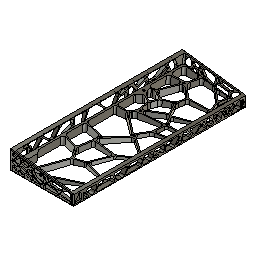
KEYBOARD CASE HOLY60 v20 - reduced size (Autodesk Fusion 360 design; units mm, degrees)
Autodesk Fusion 360 part; units mm, degrees
(part 1 of 5)
sketch "Sketch1" plane through (0, 0, 0) normal (0, 0, 1) x (1, 0, 0)
sketch "Bottom_Master" plane through (0, 0, 0) normal (0, 0, 1) x (1, 0, 0)
  line L0 (-6.9, 1.5441) -> (3.17, 1.5441)
  line L1 (3.17, 1.5441) -> (3.17, -2.18)
  line L2 (3.17, -2.18) -> (-6.9, -2.18)
  line L3 (-6.9, -2.18) -> (-6.9, 1.5441)
  line L4 (-6.7006, 1.3231) -> (2.9594, 1.3231)
  line L5 (3.0344, 1.2481) -> (3.0344, -1.9174)
  line L6 (2.9594, -1.9924) -> (-6.7006, -1.9924)
  line L7 (-6.7756, -1.9174) -> (-6.7756, 1.2481)
  line L8 (-6.6737, 0.97) -> (-6.6737, 0.6805)
  line L9 (-6.5896, 0.566) -> (-4.9141, 0.0417)
  line L10 (-4.8122, 0.054) -> (-4.3386, 0.3395)
  line L11 (-4.2652, 0.4409) -> (-4.1196, 1.0786)
  line L12 (-4.2463, 1.2375) -> (-5.5724, 1.2375)
  line L13 (-5.7409, 1.085) -> (-6.5587, 1.085)
  line L14 (-6.6737, 0.3825) -> (-6.6737, 0.3136)
  line L15 (-6.6459, 0.2188) -> (-5.3035, -1.8653)
  line L16 (-5.2194, -1.9111) -> (-4.9455, -1.9111)
  line L17 (-4.8222, -1.8065) -> (-4.628, -0.634)
  line L18 (-4.6398, -0.5466) -> (-4.8436, -0.1054)
  line L19 (-4.935, -0.0251) -> (-6.5439, 0.4779)
  line L20 (-6.5487, -1.9111) -> (-5.583, -1.9111)
  line L21 (-5.4781, -1.7181) -> (-6.4898, -0.1565)
  line L22 (-6.6737, -0.2109) -> (-6.6737, -1.7861)
  line L23 (-4.0329, 1.1248) -> (-4.1711, 0.5196)
  line L24 (-4.0646, 0.3677) -> (-3.11, 0.249)
  line L25 (-2.9431, 0.3758) -> (-2.8362, 1.0941)
  line L26 (-2.9598, 1.2375) -> (-3.8915, 1.2375)
  line L27 (-3.3566, 0.1098) -> (-3.372, -0.8279)
  line L28 (-3.5043, -0.9209) -> (-4.4494, -0.5985)
  line L29 (-4.5941, -0.4701) -> (-4.7474, -0.1509)
  line L30 (-4.6899, 0.0422) -> (-4.3293, 0.2609)
  line L31 (-4.1257, 0.3051) -> (-3.4581, 0.2259)
  line L32 (-4.7377, -1.7366) -> (-4.5829, -0.8022)
  line L33 (-4.386, -0.6849) -> (-3.406, -1.0231)
  line L34 (-3.3306, -1.0741) -> (-2.7509, -1.7458)
  line L35 (-2.8266, -1.9111) -> (-4.5897, -1.9111)
  line L36 (-3.2843, 0.055) -> (-3.3074, -0.9017)
  line L37 (-3.2468, -1.0711) -> (-2.7111, -1.6917)
  line L38 (-2.5519, -1.6814) -> (-1.9832, -0.8174)
  line L39 (-2.0116, -0.6495) -> (-3.0673, 0.159)
  line L40 (-2.4221, -1.9111) -> (-0.9115, -1.9111)
  line L41 (-0.8171, -1.7781) -> (-1.0763, -1.038)
  line L42 (-1.2125, -0.883) -> (-1.6826, -0.6472)
  line L43 (-1.8114, -0.6822) -> (-2.506, -1.7568)
  line L44 (-2.7588, 1.1526) -> (-2.8964, 0.2481)
  line L45 (-2.8298, 0.0829) -> (-2.0545, -0.5108)
  line L46 (-1.844, -0.4826) -> (-1.0421, 0.5699)
  line L47 (-1.0128, 0.6809) -> (-1.0765, 1.151)
  line L48 (-1.1756, 1.2375) -> (-2.6599, 1.2375)
  line L49 (-1.7139, -0.4217) -> (-1.0337, 0.4797)
  line L50 (-0.8469, 0.5235) -> (-0.8067, 0.5034)
  line L51 (-0.6744, 0.3335) -> (-0.4266, -0.7946)
  line L52 (-0.5312, -0.9158) -> (-0.9621, -0.886)
  line L53 (-1.1506, -0.8346) -> (-1.6786, -0.5714)
  line L54 (-1.0042, 1.1237) -> (-0.9435, 0.6879)
  line L55 (-0.8849, 0.6103) -> (-0.6399, 0.5018)
  line L56 (-0.4319, 0.4739) -> (0.07, 0.55)
  line L57 (0.1435, 0.6023) -> (0.2875, 0.8759)
  line L58 (0.2734, 0.9893) -> (0.0798, 1.2044)
  line L59 (0.0055, 1.2375) -> (-0.9051, 1.2375)
  line L60 (-0.2039, -0.8893) -> (0.1423, -0.7041)
  line L61 (0.1804, -0.5152) -> (-0.3761, 0.1713)
  line L62 (-0.5513, 0.0866) -> (-0.3486, -0.8229)
  line L63 (-0.9801, -1.0993) -> (-0.7174, -1.8444)
  line L64 (-0.623, -1.9111) -> (-0.3593, -1.9111)
  line L65 (-0.2597, -1.8022) -> (-0.3232, -1.0905)
  line L66 (-0.4156, -0.9996) -> (-0.8786, -0.9663)
  line L67 (-0.2606, -1.0975) -> (-0.1788, -1.8223)
  line L68 (-0.0794, -1.9111) -> (0.664, -1.9111)
  line L69 (0.7516, -1.7627) -> (0.2395, -0.8361)
  line L70 (0.1052, -0.7961) -> (-0.1818, -0.9482)
  arc A0 (-6.6737, 0.6805) -> (-6.5896, 0.566) centre (-6.5537, 0.6805) ccw
  arc A1 (-6.5587, 1.085) -> (-6.6737, 0.97) centre (-6.5587, 0.97) ccw
  arc A2 (-4.9141, 0.0417) -> (-4.8122, 0.054) centre (-4.8768, 0.161) ccw
  arc A3 (-4.3386, 0.3395) -> (-4.2652, 0.4409) centre (-4.4212, 0.4765) ccw
  arc A4 (-4.1196, 1.0786) -> (-4.2463, 1.2375) centre (-4.2463, 1.1075) ccw
  arc A5 (-3.8915, 1.2375) -> (-4.0329, 1.1248) centre (-3.8915, 1.0925) ccw
  arc A6 (-4.1711, 0.5196) -> (-4.0646, 0.3677) centre (-4.0492, 0.4918) ccw
  arc A7 (-4.1257, 0.3051) -> (-4.3293, 0.2609) centre (-4.1634, -0.0127) ccw
  arc A8 (-3.3566, 0.1098) -> (-3.4581, 0.2259) centre (-3.4716, 0.1117) ccw
  arc A9 (-3.0673, 0.159) -> (-3.2843, 0.055) centre (-3.1493, 0.0518) ccw
  arc A10 (-3.5043, -0.9209) -> (-3.372, -0.8279) centre (-3.472, -0.8262) ccw
  arc A11 (-3.3074, -0.9017) -> (-3.2468, -1.0711) centre (-3.0575, -0.9077) ccw
  arc A12 (-3.3306, -1.0741) -> (-3.406, -1.0231) centre (-3.4631, -1.1885) ccw
  arc A13 (-2.7111, -1.6917) -> (-2.5519, -1.6814) centre (-2.6354, -1.6264) ccw
  arc A14 (-2.8266, -1.9111) -> (-2.7509, -1.7458) centre (-2.8266, -1.8111) ccw
  arc A15 (-2.506, -1.7568) -> (-2.4221, -1.9111) centre (-2.4221, -1.8111) ccw
  arc A16 (-6.5439, 0.4779) -> (-6.6737, 0.3825) centre (-6.5737, 0.3825) ccw
  arc A17 (-6.6737, 0.3136) -> (-6.6459, 0.2188) centre (-6.4987, 0.3136) ccw
  arc A18 (-6.4898, -0.1565) -> (-6.6737, -0.2109) centre (-6.5737, -0.2109) ccw
  arc A19 (-6.6737, -1.7861) -> (-6.5487, -1.9111) centre (-6.5487, -1.7861) ccw
  arc A20 (-5.583, -1.9111) -> (-5.4781, -1.7181) centre (-5.583, -1.7861) ccw
  arc A21 (-5.3035, -1.8653) -> (-5.2194, -1.9111) centre (-5.2194, -1.8111) ccw
  arc A22 (-4.9455, -1.9111) -> (-4.8222, -1.8065) centre (-4.9455, -1.7861) ccw
  arc A23 (-4.628, -0.634) -> (-4.6398, -0.5466) centre (-4.776, -0.6095) ccw
  arc A24 (-4.8436, -0.1054) -> (-4.935, -0.0251) centre (-4.9798, -0.1683) ccw
  arc A25 (-4.6899, 0.0422) -> (-4.7474, -0.1509) centre (-4.6121, -0.086) ccw
  arc A26 (-4.5941, -0.4701) -> (-4.4494, -0.5985) centre (-4.3687, -0.3619) ccw
  arc A27 (-4.386, -0.6849) -> (-4.5829, -0.8022) centre (-4.4349, -0.8267) ccw
  arc A28 (-4.7377, -1.7366) -> (-4.5897, -1.9111) centre (-4.5897, -1.7611) ccw
  arc A29 (-2.8362, 1.0941) -> (-2.9598, 1.2375) centre (-2.9598, 1.1125) ccw
  arc A30 (-3.11, 0.249) -> (-2.9431, 0.3758) centre (-3.0915, 0.3978) ccw
  arc A31 (-2.6599, 1.2375) -> (-2.7588, 1.1526) centre (-2.6599, 1.1375) ccw
  arc A32 (-2.8964, 0.2481) -> (-2.8298, 0.0829) centre (-2.7234, 0.2218) ccw
  arc A33 (-2.0545, -0.5108) -> (-1.844, -0.4826) centre (-1.9633, -0.3917) ccw
  arc A34 (-1.0421, 0.5699) -> (-1.0128, 0.6809) centre (-1.1614, 0.6608) ccw
  arc A35 (-0.9435, 0.6879) -> (-0.8849, 0.6103) centre (-0.8444, 0.7017) ccw
  arc A36 (-1.0765, 1.151) -> (-1.1756, 1.2375) centre (-1.1756, 1.1375) ccw
  arc A37 (-0.9051, 1.2375) -> (-1.0042, 1.1237) centre (-0.9051, 1.1375) ccw
  arc A38 (-0.6399, 0.5018) -> (-0.4319, 0.4739) centre (-0.4881, 0.8447) ccw
  arc A39 (0.07, 0.55) -> (0.1435, 0.6023) centre (0.055, 0.6488) ccw
  arc A40 (0.2875, 0.8759) -> (0.2734, 0.9893) centre (0.1991, 0.9224) ccw
  arc A41 (0.0798, 1.2044) -> (0.0055, 1.2375) centre (0.0055, 1.1375) ccw
  arc A42 (-0.3761, 0.1713) -> (-0.5513, 0.0866) centre (-0.4537, 0.1084) ccw
  arc A43 (-0.3486, -0.8229) -> (-0.2039, -0.8893) centre (-0.251, -0.8012) ccw
  arc A44 (0.1423, -0.7041) -> (0.1804, -0.5152) centre (0.0833, -0.5939) ccw
  arc A45 (-0.6744, 0.3335) -> (-0.8067, 0.5034) centre (-0.9186, 0.2798) ccw
  arc A46 (-0.8469, 0.5235) -> (-1.0337, 0.4797) centre (-0.914, 0.3894) ccw
  arc A47 (-0.5312, -0.9158) -> (-0.4266, -0.7946) centre (-0.5242, -0.8161) ccw
  arc A48 (-1.1506, -0.8346) -> (-0.9621, -0.886) centre (-0.9275, -0.3872) ccw
  arc A49 (-1.7139, -0.4217) -> (-1.6786, -0.5714) centre (-1.634, -0.4819) ccw
  arc A50 (-1.9832, -0.8174) -> (-2.0116, -0.6495) centre (-2.0876, -0.7487) ccw
  arc A51 (-1.6826, -0.6472) -> (-1.8114, -0.6822) centre (-1.7274, -0.7365) ccw
  arc A52 (-1.0763, -1.038) -> (-1.2125, -0.883) centre (-1.3358, -1.1288) ccw
  arc A53 (-0.9115, -1.9111) -> (-0.8171, -1.7781) centre (-0.9115, -1.8111) ccw
  arc A54 (-0.7174, -1.8444) -> (-0.623, -1.9111) centre (-0.623, -1.8111) ccw
  arc A55 (-0.3593, -1.9111) -> (-0.2597, -1.8022) centre (-0.3593, -1.8111) ccw
  arc A56 (-0.8786, -0.9663) -> (-0.9801, -1.0993) centre (-0.8858, -1.066) ccw
  arc A57 (-0.3232, -1.0905) -> (-0.4156, -0.9996) centre (-0.4228, -1.0994) ccw
  arc A58 (-0.1818, -0.9482) -> (-0.2606, -1.0975) centre (-0.1116, -1.0807) ccw
  arc A59 (0.2395, -0.8361) -> (0.1052, -0.7961) centre (0.152, -0.8845) ccw
  arc A60 (-0.1788, -1.8223) -> (-0.0794, -1.9111) centre (-0.0794, -1.8111) ccw
  arc A61 (0.664, -1.9111) -> (0.7516, -1.7627) centre (0.664, -1.8111) ccw
  line L71 (0.3529, -0.4915) -> (0.8206, -0.26)
  line L72 (0.8626, -0.1198) -> (0.6539, 0.2361)
  line L73 (0.5098, 0.3558) -> (0.2183, 0.4607)
  line L74 (0.0544, 0.4784) -> (-0.3024, 0.4317)
  line L75 (-0.367, 0.2694) -> (0.231, -0.465)
  line L76 (0.2751, -0.7557) -> (0.8648, -1.8331)
  line L77 (0.9964, -1.9111) -> (1.4354, -1.9111)
  line L78 (1.5778, -1.8081) -> (1.6526, -1.5814)
  line L79 (1.6707, -1.376) -> (1.5399, -0.4704)
  line L80 (1.4184, -0.3443) -> (1.0937, -0.285)
  line L81 (0.8584, -0.3186) -> (0.3288, -0.5839)
  line L82 (1.6507, -1.8105) -> (1.7201, -1.619)
  line L83 (1.8608, -1.4822) -> (2.3053, -1.3346)
  line L84 (2.3496, -1.3303) -> (2.8214, -1.3912)
  line L85 (2.9304, -1.5152) -> (2.9304, -1.8111)
  line L86 (2.8304, -1.9111) -> (1.7212, -1.9111)
  line L87 (2.9304, -1.2524) -> (2.9304, -0.8256)
  line L88 (2.7974, -0.778) -> (2.4806, -1.1638)
  line L89 (2.5289, -1.2857) -> (2.8457, -1.3268)
  line L90 (1.6012, -0.4606) -> (1.7323, -1.3326)
  line L91 (1.8627, -1.4127) -> (2.2639, -1.2798)
  line L92 (2.3326, -1.2326) -> (2.8849, -0.56)
  line L93 (2.9304, -0.4331) -> (2.9304, 0.0812)
  line L94 (2.8125, 0.2278) -> (2.3736, 0.324)
  line L95 (2.1106, 0.2397) -> (1.6629, -0.2558)
  line L96 (0.6623, 0.4857) -> (0.8052, 0.7474)
  line L97 (0.8235, 0.97) -> (0.803, 1.0285)
  line L98 (0.6588, 1.0822) -> (0.4617, 0.9689)
  line L99 (0.3453, 0.8476) -> (0.242, 0.6497)
  line L100 (0.2951, 0.51) -> (0.5081, 0.4288)
  line L101 (0.715, 0.4334) -> (0.8673, 0.7159)
  line L102 (1.0156, 0.7755) -> (1.9066, 0.4891)
  line L103 (1.9929, 0.3806) -> (1.9978, 0.3231)
  line L104 (1.9501, 0.1758) -> (1.6045, -0.2261)
  line L105 (1.4372, -0.2835) -> (1.0557, -0.2067)
  line L106 (0.9566, -0.1367) -> (0.7189, 0.2605)
  line L107 (0.8585, 1.0695) -> (0.9096, 0.9299)
  line L108 (0.989, 0.8538) -> (1.935, 0.5517)
  line L109 (2.0966, 0.6895) -> (2.0328, 1.11)
  line L110 (1.8845, 1.2375) -> (0.9758, 1.2375)
  line L111 (2.1178, 1.0629) -> (2.2109, 0.5032)
  line L112 (2.286, 0.4225) -> (2.745, 0.3112)
  line L113 (2.9304, 0.4569) -> (2.9304, 1.0875)
  line L114 (2.7804, 1.2375) -> (2.2658, 1.2375)
  arc A62 (-0.3024, 0.4317) -> (-0.367, 0.2694) centre (-0.2894, 0.3326) ccw
  arc A63 (0.231, -0.465) -> (0.3529, -0.4915) centre (0.3085, -0.4019) ccw
  arc A64 (0.8206, -0.26) -> (0.8626, -0.1198) centre (0.7763, -0.1704) ccw
  arc A65 (0.6539, 0.2361) -> (0.5098, 0.3558) centre (0.4167, 0.0971) ccw
  arc A66 (0.2183, 0.4607) -> (0.0544, 0.4784) centre (0.0998, 0.1313) ccw
  arc A67 (0.242, 0.6497) -> (0.2951, 0.51) centre (0.3307, 0.6034) ccw
  arc A68 (0.4617, 0.9689) -> (0.3453, 0.8476) centre (0.6113, 0.7088) ccw
  arc A69 (0.803, 1.0285) -> (0.6588, 1.0822) centre (0.7086, 0.9955) ccw
  arc A70 (0.8052, 0.7474) -> (0.8235, 0.97) centre (0.5639, 0.8792) ccw
  arc A71 (0.5081, 0.4288) -> (0.6623, 0.4857) centre (0.5526, 0.5456) ccw
  arc A72 (0.9758, 1.2375) -> (0.8585, 1.0695) centre (0.9758, 1.1125) ccw
  arc A73 (0.9096, 0.9299) -> (0.989, 0.8538) centre (1.027, 0.9729) ccw
  arc A74 (2.0328, 1.11) -> (1.8845, 1.2375) centre (1.8845, 1.0875) ccw
  arc A75 (1.935, 0.5517) -> (2.0966, 0.6895) centre (1.973, 0.6708) ccw
  arc A76 (1.0156, 0.7755) -> (0.8673, 0.7159) centre (0.9773, 0.6565) ccw
  arc A77 (0.715, 0.4334) -> (0.7189, 0.2605) centre (0.869, 0.3504) ccw
  arc A78 (0.9566, -0.1367) -> (1.0557, -0.2067) centre (1.0853, -0.0596) ccw
  arc A79 (1.4372, -0.2835) -> (1.6045, -0.2261) centre (1.4718, -0.1119) ccw
  arc A80 (1.9929, 0.3806) -> (1.9066, 0.4891) centre (1.8684, 0.3701) ccw
  arc A81 (1.9501, 0.1758) -> (1.9978, 0.3231) centre (1.7985, 0.3062) ccw
  arc A82 (0.3288, -0.5839) -> (0.2751, -0.7557) centre (0.3847, -0.6956) ccw
  arc A83 (1.0937, -0.285) -> (0.8584, -0.3186) centre (1.0263, -0.6539) ccw
  arc A84 (1.5399, -0.4704) -> (1.4184, -0.3443) centre (1.3914, -0.4919) ccw
  arc A85 (0.8648, -1.8331) -> (0.9964, -1.9111) centre (0.9964, -1.7611) ccw
  arc A86 (1.4354, -1.9111) -> (1.5778, -1.8081) centre (1.4354, -1.7611) ccw
  arc A87 (1.6526, -1.5814) -> (1.6707, -1.376) centre (1.2253, -1.4404) ccw
  arc A88 (1.7323, -1.3326) -> (1.8627, -1.4127) centre (1.8312, -1.3178) ccw
  arc A89 (2.2639, -1.2798) -> (2.3326, -1.2326) centre (2.2167, -1.1374) ccw
  arc A90 (1.6629, -0.2558) -> (1.6012, -0.4606) centre (1.8484, -0.4234) ccw
  arc A91 (2.3736, 0.324) -> (2.1106, 0.2397) centre (2.3147, 0.0554) ccw
  arc A92 (2.9304, 0.0812) -> (2.8125, 0.2278) centre (2.7804, 0.0812) ccw
  arc A93 (2.8849, -0.56) -> (2.9304, -0.4331) centre (2.7304, -0.4331) ccw
  arc A94 (1.8608, -1.4822) -> (1.7201, -1.619) centre (1.9317, -1.6957) ccw
  arc A95 (2.3496, -1.3303) -> (2.3053, -1.3346) centre (2.3368, -1.4295) ccw
  arc A96 (2.9304, -1.5152) -> (2.8214, -1.3912) centre (2.8054, -1.5152) ccw
  arc A97 (2.8304, -1.9111) -> (2.9304, -1.8111) centre (2.8304, -1.8111) ccw
  arc A98 (1.6507, -1.8105) -> (1.7212, -1.9111) centre (1.7212, -1.8361) ccw
  arc A99 (2.9304, -0.8256) -> (2.7974, -0.778) centre (2.8554, -0.8256) ccw
  arc A100 (2.4806, -1.1638) -> (2.5289, -1.2857) centre (2.5386, -1.2114) ccw
  arc A101 (2.8457, -1.3268) -> (2.9304, -1.2524) centre (2.8554, -1.2524) ccw
  arc A102 (2.2658, 1.2375) -> (2.1178, 1.0629) centre (2.2658, 1.0875) ccw
  arc A103 (2.2109, 0.5032) -> (2.286, 0.4225) centre (2.3096, 0.5196) ccw
  arc A104 (2.745, 0.3112) -> (2.9304, 0.4569) centre (2.7804, 0.4569) ccw
  arc A105 (2.9304, 1.0875) -> (2.7804, 1.2375) centre (2.7804, 1.0875) ccw
  spline S0 degree 5 poles (-5.7409, 1.085) (-5.7331, 1.0864) (-5.719, 1.0897) (-5.702, 1.0963) (-5.6871, 1.108) (-5.6778, 1.1266) (-5.6732, 1.1474) (-5.6689, 1.1688) (-5.6612, 1.1892) (-5.6484, 1.2074) (-5.6295, 1.2223) (-5.6096, 1.2308) (-5.592, 1.235) (-5.5791, 1.2369) (-5.5724, 1.2375) knots 0 0 0 0 0 0 0.1 0.2 0.3 0.4 0.5 0.6 0.7 0.8 0.9 1 1 1 1 1 1
  line L115 (-5.7795, 1.078) -> (-5.7023, 1.0919)
  line L116 (-5.6052, 1.2343) -> (-5.5396, 1.2408)
  arc A106 (-6.7006, 1.3231) -> (-6.7756, 1.2481) centre (-6.7006, 1.2481) ccw
  arc A107 (-6.7756, -1.9174) -> (-6.7006, -1.9924) centre (-6.7006, -1.9174) ccw
  arc A108 (2.9594, -1.9924) -> (3.0344, -1.9174) centre (2.9594, -1.9174) ccw
  arc A109 (3.0344, 1.2481) -> (2.9594, 1.3231) centre (2.9594, 1.2481) ccw
  point P0 (-5.6681, 1.1684)
  dimension "d1" = 0.12
  dimension "d2" = 0.115
  dimension "d3" = 0.125
  dimension "d4" = 0.16
  dimension "d5" = 0.13
  dimension "d6" = 0.145
  dimension "d7" = 0.125
  dimension "d8" = 0.32
  dimension "d9" = 0.115
  dimension "d10" = 0.135
  dimension "d11" = 0.1
  dimension "d12" = 0.25
  dimension "d13" = 0.175
  dimension "d14" = 0.1
  dimension "d15" = 0.1
  dimension "d16" = 0.1
  dimension "d17" = 0.1
  dimension "d18" = 0.175
  dimension "d19" = 0.1
  dimension "d20" = 0.125
  dimension "d21" = 0.125
  dimension "d22" = 0.1
  dimension "d23" = 0.125
  dimension "d24" = 0.15
  dimension "d25" = 0.15
  dimension "d26" = 0.15
  dimension "d27" = 0.25
  dimension "d28" = 0.15
  dimension "d29" = 0.15
  dimension "d30" = 0.125
  dimension "d31" = 0.15
  dimension "d32" = 0.1
  dimension "d33" = 0.175
  dimension "d34" = 0.15
  dimension "d35" = 0.15
  dimension "d36" = 0.1
  dimension "d37" = 0.1
  dimension "d38" = 0.1
  dimension "d39" = 0.375
  dimension "d40" = 0.1
  dimension "d41" = 0.1
  dimension "d42" = 0.1
  dimension "d43" = 0.1
  dimension "d44" = 0.1
  dimension "d45" = 0.125
  dimension "d46" = 0.25
  dimension "d47" = 0.15
  dimension "d48" = 0.1
  dimension "d49" = 0.5
  dimension "d50" = 0.1
  dimension "d51" = 0.125
  dimension "d52" = 0.1
  dimension "d53" = 0.275
  dimension "d54" = 0.1
  dimension "d55" = 0.1
  dimension "d56" = 0.1
  dimension "d57" = 0.1
  dimension "d58" = 0.1
  dimension "d59" = 0.15
  dimension "d60" = 0.1
  dimension "d61" = 0.1
  dimension "d62" = 0.1
  dimension "d63" = 0.1
  dimension "d64" = 0.1
  dimension "d65" = 0.1
  dimension "d66" = 0.275
  dimension "d67" = 0.35
  dimension "d68" = 0.1
  dimension "d69" = 0.3
  dimension "d70" = 0.1
  dimension "d71" = 0.275
  dimension "d72" = 0.125
  dimension "d73" = 0.125
  dimension "d74" = 0.125
  dimension "d75" = 0.15
  dimension "d76" = 0.125
  dimension "d77" = 0.125
  dimension "d78" = 0.175
  dimension "d79" = 0.15
  dimension "d80" = 0.175
  dimension "d81" = 0.125
  dimension "d82" = 0.2
  dimension "d83" = 0.125
  dimension "d84" = 0.375
  dimension "d85" = 0.15
  dimension "d86" = 0.15
  dimension "d87" = 0.15
  dimension "d88" = 0.45
  dimension "d89" = 0.1
  dimension "d90" = 0.15
  dimension "d91" = 0.25
  dimension "d92" = 0.275
  dimension "d93" = 0.15
  dimension "d94" = 0.2
  dimension "d95" = 0.225
  dimension "d96" = 0.1
  dimension "d97" = 0.125
  dimension "d98" = 0.1
  dimension "d99" = 0.075
  dimension "d100" = 0.075
  dimension "d101" = 0.075
  dimension "d102" = 0.075
  dimension "d103" = 0.15
  dimension "d104" = 0.1
  dimension "d105" = 0.15
  dimension "d106" = 0.15
  dimension "d107" = 0.075
  constraint horizontal L0
  constraint vertical L1
  constraint horizontal L2
  constraint vertical L3
  constraint horizontal L4
  constraint vertical L5
  constraint horizontal L6
  constraint vertical L7
  constraint vertical L8
  constraint horizontal L12
  constraint parallel L7 L14
  constraint perpendicular L7 L16
  constraint horizontal L20
  constraint perpendicular L20 L22
  constraint parallel L11 L23
  constraint parallel L17 L32
  constraint parallel L34 L37
  constraint parallel L6 L40
  constraint parallel L39 L45
  constraint horizontal L64
  constraint horizontal L68
  constraint tangent L8 A0
  constraint tangent L9 A0
  constraint tangent L8 A1
  constraint tangent L13 A1
  constraint tangent L9 A2
  constraint tangent L10 A2
  constraint tangent L10 A3
  constraint tangent L11 A3
  constraint tangent L11 A4
  constraint tangent L12 A4
  constraint tangent L23 A5
  constraint tangent L26 A5
  constraint tangent L23 A6
  constraint tangent L24 A6
  constraint tangent L30 A7
  constraint tangent L31 A7
  constraint tangent L27 A8
  constraint tangent L31 A8
  constraint tangent L39 A9
  constraint tangent L36 A9
  constraint tangent L27 A10
  constraint tangent L28 A10
  constraint tangent L36 A11
  constraint tangent L37 A11
  constraint tangent L33 A12
  constraint tangent L34 A12
  constraint tangent L37 A13
  constraint tangent L38 A13
  constraint tangent L34 A14
  constraint tangent L35 A14
  constraint tangent L40 A15
  constraint tangent L43 A15
  constraint tangent L14 A16
  constraint tangent L19 A16
  constraint tangent L14 A17
  constraint tangent L15 A17
  constraint tangent L21 A18
  constraint tangent L22 A18
  constraint tangent L20 A19
  constraint tangent L22 A19
  constraint tangent L20 A20
  constraint tangent L21 A20
  constraint tangent L15 A21
  constraint tangent L16 A21
  constraint tangent L16 A22
  constraint tangent L17 A22
  constraint tangent L17 A23
  constraint tangent L18 A23
  constraint tangent L18 A24
  constraint tangent L19 A24
  constraint tangent L29 A25
  constraint tangent L30 A25
  constraint tangent L28 A26
  constraint tangent L29 A26
  constraint tangent L32 A27
  constraint tangent L33 A27
  constraint tangent L32 A28
  constraint tangent L35 A28
  constraint tangent L25 A29
  constraint tangent L26 A29
  constraint tangent L24 A30
  constraint tangent L25 A30
  constraint tangent L44 A31
  constraint tangent L48 A31
  constraint tangent L44 A32
  constraint tangent L45 A32
  constraint tangent L45 A33
  constraint tangent L46 A33
  constraint tangent L46 A34
  constraint tangent L47 A34
  constraint tangent L54 A35
  constraint tangent L55 A35
  constraint tangent L47 A36
  constraint tangent L48 A36
  constraint tangent L54 A37
  constraint tangent L59 A37
  constraint tangent L55 A38
  constraint tangent L56 A38
  constraint tangent L56 A39
  constraint tangent L57 A39
  constraint tangent L57 A40
  constraint tangent L58 A40
  constraint tangent L58 A41
  constraint tangent L59 A41
  constraint tangent L62 A42
  constraint tangent L61 A42
  constraint tangent L60 A43
  constraint tangent L62 A43
  constraint tangent L60 A44
  constraint tangent L61 A44
  constraint tangent L50 A45
  constraint tangent L51 A45
  constraint tangent L49 A46
  constraint tangent L50 A46
  constraint tangent L51 A47
  constraint tangent L52 A47
  constraint tangent L52 A48
  constraint tangent L53 A48
  constraint tangent L49 A49
  constraint tangent L53 A49
  constraint tangent L38 A50
  constraint tangent L39 A50
  constraint tangent L42 A51
  constraint tangent L43 A51
  constraint tangent L41 A52
  constraint tangent L42 A52
  constraint tangent L40 A53
  constraint tangent L41 A53
  constraint tangent L63 A54
  constraint tangent L64 A54
  constraint tangent L64 A55
  constraint tangent L65 A55
  constraint tangent L63 A56
  constraint tangent L66 A56
  constraint tangent L65 A57
  constraint tangent L66 A57
  constraint tangent L67 A58
  constraint tangent L70 A58
  constraint tangent L69 A59
  constraint tangent L70 A59
  constraint tangent L67 A60
  constraint tangent L68 A60
  constraint tangent L68 A61
  constraint tangent L69 A61
  constraint horizontal L86
  constraint parallel L5 L87
  constraint parallel L88 L92
  constraint vertical L93
  constraint tangent L74 A62
  constraint tangent L75 A62
  constraint tangent L71 A63
  constraint tangent L75 A63
  constraint tangent L71 A64
  constraint tangent L72 A64
  constraint tangent L72 A65
  constraint tangent L73 A65
  constraint tangent L73 A66
  constraint tangent L74 A66
  constraint tangent L99 A67
  constraint tangent L100 A67
  constraint tangent L98 A68
  constraint tangent L99 A68
  constraint tangent L98 A69
  constraint tangent L97 A69
  constraint tangent L96 A70
  constraint tangent L97 A70
  constraint tangent L96 A71
  constraint tangent L100 A71
  constraint tangent L107 A72
  constraint tangent L110 A72
  constraint tangent L107 A73
  constraint tangent L108 A73
  constraint tangent L109 A74
  constraint tangent L110 A74
  constraint tangent L108 A75
  constraint tangent L109 A75
  constraint tangent L101 A76
  constraint tangent L102 A76
  constraint tangent L101 A77
  constraint tangent L106 A77
  constraint tangent L105 A78
  constraint tangent L106 A78
  constraint tangent L104 A79
  constraint tangent L105 A79
  constraint tangent L102 A80
  constraint tangent L103 A80
  constraint tangent L103 A81
  constraint tangent L104 A81
  constraint tangent L76 A82
  constraint tangent L81 A82
  constraint tangent L80 A83
  constraint tangent L81 A83
  constraint tangent L79 A84
  constraint tangent L80 A84
  constraint tangent L76 A85
  constraint tangent L77 A85
  constraint tangent L77 A86
  constraint tangent L78 A86
  constraint tangent L78 A87
  constraint tangent L79 A87
  constraint tangent L90 A88
  constraint tangent L91 A88
  constraint tangent L91 A89
  constraint tangent L92 A89
  constraint tangent L90 A90
  constraint tangent L95 A90
  constraint tangent L94 A91
  constraint tangent L95 A91
  constraint tangent L93 A92
  constraint tangent L94 A92
  constraint tangent L92 A93
  constraint tangent L93 A93
  constraint tangent L82 A94
  constraint tangent L83 A94
  constraint tangent L83 A95
  constraint tangent L84 A95
  constraint tangent L84 A96
  constraint tangent L85 A96
  constraint tangent L85 A97
  constraint tangent L86 A97
  constraint tangent L82 A98
  constraint tangent L86 A98
  constraint tangent L87 A99
  constraint tangent L88 A99
  constraint tangent L88 A100
  constraint tangent L89 A100
  constraint tangent L87 A101
  constraint tangent L89 A101
  constraint tangent L111 A102
  constraint tangent L114 A102
  constraint tangent L111 A103
  constraint tangent L112 A103
  constraint tangent L112 A104
  constraint tangent L113 A104
  constraint tangent L113 A105
  constraint tangent L114 A105
  constraint midpoint L13.start L115
  constraint midpoint L12.end L116
  constraint collinear L12 L26
  constraint collinear L26 L48
  constraint collinear L48 L59
  constraint collinear L59 L110
  constraint collinear L110 L114
  constraint collinear L93 L113
  constraint collinear L87 L93
  constraint collinear L85 L87
  constraint collinear L77 L86
  constraint collinear L68 L77
  constraint collinear L64 L68
  constraint collinear L40 L64
  constraint collinear L35 L40
  constraint collinear L16 L35
  constraint collinear L16 L20
  constraint collinear L14 L22
  constraint collinear L8 L14
  constraint tangent L7 A106
  constraint tangent L4 A106
  constraint tangent L6 A107
  constraint tangent L7 A107
  constraint equal A106 A107
  constraint tangent L5 A108
  constraint tangent L6 A108
  constraint equal A106 A108
  constraint tangent L4 A109
  constraint tangent L5 A109
  constraint equal A106 A109
  measures "d1" radius of A0
  measures "d2" radius of A1
  measures "d3" radius of A2
  measures "d4" radius of A3
  measures "d5" radius of A4
  measures "d6" radius of A5
  measures "d7" radius of A6
  measures "d8" radius of A7
  measures "d9" radius of A8
  measures "d10" radius of A9
  measures "d11" radius of A10
  measures "d12" radius of A11
  measures "d13" radius of A12
  measures "d14" radius of A13
  measures "d15" radius of A14
  measures "d16" radius of A15
  measures "d17" radius of A16
  measures "d18" radius of A17
  measures "d19" radius of A18
  measures "d20" radius of A19
  measures "d21" radius of A20
  measures "d22" radius of A21
  measures "d23" radius of A22
  measures "d24" radius of A23
  measures "d25" radius of A24
  measures "d26" radius of A25
  measures "d27" radius of A26
  measures "d28" radius of A27
  measures "d29" radius of A28
  measures "d30" radius of A29
  measures "d31" radius of A30
  measures "d32" radius of A31
  measures "d33" radius of A32
  measures "d34" radius of A33
  measures "d35" radius of A34
  measures "d36" radius of A35
  measures "d37" radius of A36
  measures "d38" radius of A37
  measures "d39" radius of A38
  measures "d40" radius of A39
  measures "d41" radius of A40
  measures "d42" radius of A41
  measures "d43" radius of A42
  measures "d44" radius of A43
  measures "d45" radius of A44
  measures "d46" radius of A45
  measures "d47" radius of A46
  measures "d48" radius of A47
  measures "d49" radius of A48
  measures "d50" radius of A49
  measures "d51" radius of A50
  measures "d52" radius of A51
  measures "d53" radius of A52
  measures "d54" radius of A53
  measures "d55" radius of A54
  measures "d56" radius of A55
  measures "d57" radius of A56
  measures "d58" radius of A57
  measures "d59" radius of A58
  measures "d60" radius of A59
  measures "d61" radius of A60
  measures "d62" radius of A61
  measures "d63" radius of A62
  measures "d64" radius of A63
  measures "d65" radius of A64
  measures "d66" radius of A65
  measures "d67" radius of A66
  measures "d68" radius of A67
  measures "d69" radius of A68
  measures "d70" radius of A69
  measures "d71" radius of A70
  measures "d72" radius of A71
  measures "d73" radius of A72
  measures "d74" radius of A73
  measures "d75" radius of A74
  measures "d76" radius of A75
  measures "d77" radius of A76
  measures "d78" radius of A77
  measures "d79" radius of A78
  measures "d80" radius of A79
  measures "d81" radius of A80
  measures "d82" radius of A81
  measures "d83" radius of A82
  measures "d84" radius of A83
  measures "d85" radius of A84
  measures "d86" radius of A85
  measures "d87" radius of A86
  measures "d88" radius of A87
  measures "d89" radius of A88
  measures "d90" radius of A89
  measures "d91" radius of A90
  measures "d92" radius of A91
  measures "d93" radius of A92
  measures "d94" radius of A93
  measures "d95" radius of A94
  measures "d96" radius of A95
  measures "d97" radius of A96
  measures "d98" radius of A97
  measures "d99" radius of A98
  measures "d100" radius of A99
  measures "d101" radius of A100
  measures "d102" radius of A101
  measures "d103" radius of A102
  measures "d104" radius of A103
  measures "d105" radius of A104
  measures "d106" radius of A105
  measures "d107" radius of A106
sketch "Sketch3" plane through (0, 0, 0) normal (0, 0, 1) x (1, 0, 0)
  line L0 (-50.3809, 104.0983) -> (-18.0784, 104.0983)
  line L1 (-18.0784, 104.0983) -> (-18.0784, -4.9017)
  line L2 (-18.0784, -4.9017) -> (-36.6784, -4.9017)
  line L3 (-36.6784, -4.9017) -> (-50.3809, 104.0983)
  line L4 (-36.6784, -4.9017) -> (-18.0784, -2.5635)
  line L5 (-18.0784, 104.0983) -> (-49.8784, 100.1006)
  dimension "d108" = 18.6
  dimension "d109" = 109
  dimension "d110" = 31.8
  constraint perpendicular L0 L1
  constraint perpendicular L1 L2
  constraint perpendicular L3 L4
  constraint coincident L1 L4.end
  constraint coincident L3 L5.end
  constraint perpendicular L3 L5
  constraint vertical L1
  measures "d108" horizontal distance of L2.end L4.end
  measures "d109" vertical distance of L0.start L1.end
  measures "d110" horizontal distance of L0.end L5.end
sketch "Sketch4" plane through (0, 0, 0) normal (0, 1, 0) x (1, 0, 0)
  line L0 (-113.7873, -4.9975) -> (-109.7896, -36.7975)
  line L1 (-4.7873, -23.5975) -> (-113.7873, -37.3)
  line L2 (-4.7873, -4.9975) -> (-4.7873, -23.5975)
  line L3 (-113.7873, -37.3) -> (-113.7873, -4.9975)
  line L4 (-113.7873, -4.9975) -> (-4.7873, -4.9975)
  line L5 (-4.7873, -23.5975) -> (-7.1255, -4.9975)
  constraint perpendicular L3 L4
  constraint perpendicular L2 L4
  constraint perpendicular L1 L5
  constraint coincident L5.end L4
  constraint coincident L0.end L1
  constraint perpendicular L0 L1
extrude "Extrude2" add sketch "Sketch4" along normal blind 300
sketch "Sketch6" plane through (2.8458, 0, 22.6379) normal (0.12473, 0, 0.992191) x (0, 1, 0)
  line L0 (0, 117.5511) -> (0, 7.6932)
  line L1 (0, 7.6932) -> (300, 7.6932)
  line L2 (300, 7.6932) -> (300, 117.5511)
  line L3 (300, 117.5511) -> (0, 117.5511)
  line L4 (298.5325, 117.5511) -> (298.5325, 7.6901)
  line L5 (1.4675, 117.5511) -> (298.5325, 117.5511)
  line L6 (298.5325, 7.6901) -> (1.4675, 7.6901)
  line L7 (1.4675, 7.6901) -> (1.4675, 117.5511)
  line L8 (7.3501, 111.0307) -> (292.6499, 111.0307)
  arc A0 (7.3501, 111.0307) -> (5.1376, 108.8182) centre (7.3501, 108.8182) ccw
  line L9 (5.1376, 15.4368) -> (5.1376, 108.8182)
  line L10 (292.6499, 13.2243) -> (7.3501, 13.2243)
  arc A1 (5.1376, 15.4368) -> (7.3501, 13.2243) centre (7.3501, 15.4368) ccw
  arc A2 (292.6499, 13.2243) -> (294.8624, 15.4368) centre (292.6499, 15.4368) ccw
  line L11 (294.8624, 108.8182) -> (294.8624, 15.4368)
  arc A3 (294.8624, 108.8182) -> (292.6499, 111.0307) centre (292.6499, 108.8182) ccw
  dimension "d119" = 2.2125
  dimension "d120" = 109.861
  dimension "d121" = 297.065
  dimension "d122" = 3.6701
  dimension "d124" = 6.5204
  dimension "d125" = 5.5342
  dimension "d126" = 3.6701
  dimension "d127" = 1.4675
  constraint horizontal L5
  constraint vertical L4
  constraint horizontal L6
  constraint vertical L7
  constraint horizontal L8
  constraint vertical L11
  constraint horizontal L10
  constraint vertical L9
  constraint tangent A0 L9
  constraint tangent L8 A0
  constraint tangent L10 A1
  constraint tangent L9 A1
  constraint equal A0 A1
  constraint tangent A2 L11
  constraint tangent L10 A2
  constraint equal A0 A2
  constraint tangent L8 A3
  constraint tangent L11 A3
  constraint equal A0 A3
  constraint coincident L3 L5.start
  measures "d119" radius of A0
  measures "d120" distance of L5.start L6.end
  measures "d121" distance of L5.start L4.start
  measures "d122" distance of L7 L9
  measures "d124" distance of L5 L8
  measures "d125" distance of L6 L10
  measures "d126" distance of L4 L11
  measures "d127" distance of L0 L7
extrude "Extrude3" cut sketch "Sketch6" against normal blind 17 contours L8 A0 L9 L10 A1 A2 L11 A3
ref_plane "WorkPlane2" through (-109.4382, 150, 19.6195) normal (0, 0, 1) x (0, 1, 0)
sketch "Sketch11" plane through (0, 0, 19.6195) normal (0, 0, 1) x (1, 0, 0)
  point P0 (-113.7873, 1.4675)
sketch "Sketch12" plane through (0.7254, 0, 5.7707) normal (0.12473, 0, 0.992191) x (0, 1, 0)
  arc A0 (292.6499, 13.2243) -> (294.8624, 15.4368) centre (292.6499, 15.4368) ccw
  line L0 (294.8624, 15.4368) -> (294.8624, 108.8182)
  arc A1 (294.8624, 108.8182) -> (292.6499, 111.0307) centre (292.6499, 108.8182) ccw
  line L1 (5.1376, 108.8182) -> (5.1376, 15.4368)
  arc A2 (5.1376, 15.4368) -> (7.3501, 13.2243) centre (7.3501, 15.4368) ccw
  line L2 (7.3501, 13.2243) -> (292.6499, 13.2243)
  arc A3 through (273.8014, 32.0403, -0.5425) (274.9144, 32.5926, -0.5425) (275.8299, 33.4326, -0.5425)
  line L3 (253.5627, 16.4556, -0.5425) -> (255.7697, 23.1441, -0.5425)
  arc A4 through (255.7129, 16.3839, -0.5425) (255.9812, 14.3596, -0.5425) (257.7929, 13.4172, -0.5425)
  line L4 (3.4675, 115.3458, -0.5425) -> (300.5325, 115.3458, -0.5425)
  arc A5 through (249.3606, 13.4172, -0.5425) (251.9533, 14.2563, -0.5425) (253.5627, 16.4556, -0.5425)
  arc A6 through (258.1218, 30.4824, -0.5425) (259.4949, 28.4075, -0.5425) (261.9665, 28.1207, -0.5425)
  arc A7 through (294.3211, 11.019, -0.5425) (295.8856, 11.667, -0.5425) (296.5336, 13.2315, -0.5425)
  arc A8 through (290.5135, 13.4172, -0.5425) (292.5995, 14.2812, -0.5425) (293.4635, 16.3672, -0.5425)
  arc A9 through (255.7697, 23.1441, -0.5425) (256.3873, 26.142, -0.5425) (256.3019, 29.2016, -0.5425)
  line L5 (236.4115, 13.4172, -0.5425) -> (249.3606, 13.4172, -0.5425)
  line L6 (123.6315, 13.4172, -0.5425) -> (71.6211, 13.4172, -0.5425)
  arc A10 through (276.3301, 30.5509, -0.5425) (275.6694, 30.5615, -0.5425) (275.0229, 30.4248, -0.5425)
  line L7 (294.3211, 11.019, -0.5425) -> (9.3501, 11.019, -0.5425)
  line L8 (87.1104, 80.6432, -0.5425) -> (115.2719, 77.1399, -0.5425)
  line L9 (261.9665, 28.1207, -0.5425) -> (273.8014, 32.0403, -0.5425)
  line L10 (255.7129, 16.3839, -0.5425) -> (257.7618, 22.0339, -0.5425)
  arc A11 through (293.4635, 45.4408, -0.5425) (291.9967, 47.5238, -0.5425) (289.5412, 46.8449, -0.5425)
  line L11 (300.5325, 5.4848, -0.5425) -> (3.4675, 5.4848, -0.5425)
  line L12 (111.2377, 38.1979, -0.5425) -> (127.0398, 19.8883, -0.5425)
  line L13 (289.5412, 46.8449, -0.5425) -> (280.1951, 35.4638, -0.5425)
  line L14 (290.5135, 13.4172, -0.5425) -> (257.7929, 13.4172, -0.5425)
  line L15 (119.7027, 106.3021, -0.5425) -> (92.2179, 106.3021, -0.5425)
  arc A12 through (290.9668, 30.6546, -0.5425) (292.7116, 31.1869, -0.5425) (293.4635, 32.8488, -0.5425)
  line L16 (281.6207, 31.8655, -0.5425) -> (290.9668, 30.6546, -0.5425)
  arc A13 through (261.9099, 26.0704, -0.5425) (259.3727, 24.5281, -0.5425) (257.7618, 22.0339, -0.5425)
  arc A14 through (116.5331, 74.4839, -0.5425) (112.392, 74.914, -0.5425) (110.1305, 71.4182, -0.5425)
  line L17 (293.4635, 32.8488, -0.5425) -> (293.4635, 45.4408, -0.5425)
  line L18 (261.9099, 26.0704, -0.5425) -> (275.0229, 30.4248, -0.5425)
  arc A15 through (293.4635, 25.0979, -0.5425) (292.5453, 27.5328, -0.5425) (290.2479, 28.755, -0.5425)
  arc A16 through (280.1951, 35.4638, -0.5425) (279.848, 33.2447, -0.5425) (281.6207, 31.8655, -0.5425)
  line L19 (293.4635, 25.0979, -0.5425) -> (293.4635, 16.3672, -0.5425)
  line L20 (108.7653, 38.1075, -0.5425) -> (125.8648, 18.2946, -0.5425)
  line L21 (276.3301, 30.5509, -0.5425) -> (290.2479, 28.755, -0.5425)
  line L22 (9.3501, 108.8254, -0.5425) -> (294.3211, 108.8254, -0.5425)
  line L23 (207.1787, 106.3021, -0.5425) -> (180.3167, 106.3021, -0.5425)
  line L24 (81.7514, 106.3021, -0.5425) -> (42.6317, 106.3021, -0.5425)
  line L25 (70.1435, 53.6696, -0.5425) -> (64.1302, 66.6858, -0.5425)
  line L26 (107.9965, 73.0335, -0.5425) -> (107.543, 45.3729, -0.5425)
  line L27 (190.7528, 72.3495, -0.5425) -> (196.7325, 45.5183, -0.5425)
  line L28 (10.1419, 98.4088, -0.5425) -> (10.1419, 89.8693, -0.5425)
  arc A17 through (70.492, 51.0906, -0.5425) (70.5116, 52.4063, -0.5425) (70.1435, 53.6696, -0.5425)
  line L29 (10.9643, 76.2502, -0.5425) -> (50.5643, 14.7697, -0.5425)
  arc A18 through (108.7653, 38.1075, -0.5425) (107.7529, 39.0083, -0.5425) (106.5409, 39.6147, -0.5425)
  arc A19 through (195.9237, 74.8489, -0.5425) (192.3483, 75.6473, -0.5425) (190.7528, 72.3495, -0.5425)
  line L30 (194.2757, 83.7751, -0.5425) -> (209.0833, 86.0187, -0.5425)
  arc A20 through (109.448, 43.1948, -0.5425) (109.8778, 40.5298, -0.5425) (111.2377, 38.1979, -0.5425)
  line L31 (110.1305, 71.4182, -0.5425) -> (109.448, 43.1948, -0.5425)
  arc A21 through (103.6411, 42.6291, -0.5425) (106.2902, 43.0081, -0.5425) (107.543, 45.3729, -0.5425)
  arc A22 through (42.3199, 13.4172, -0.5425) (45.5596, 15.3434, -0.5425) (45.4146, 19.1097, -0.5425)
  arc A23 through (64.1302, 66.6858, -0.5425) (63.0327, 68.1552, -0.5425) (61.4337, 69.0534, -0.5425)
  arc A24 through (92.2179, 106.3021, -0.5425) (89.5511, 105.369, -0.5425) (88.0477, 102.9769, -0.5425)
  arc A25 through (67.2556, 18.5654, -0.5425) (68.2461, 14.9803, -0.5425) (71.6211, 13.4172, -0.5425)
  arc A26 through (79.0291, 79.809, -0.5425) (80.4163, 81.0843, -0.5425) (81.1941, 82.8007, -0.5425)
  line L32 (67.2556, 18.5654, -0.5425) -> (71.8221, 46.13, -0.5425)
  arc A27 through (83.9707, 85.1234, -0.5425) (84.5459, 82.1862, -0.5425) (87.1104, 80.6432, -0.5425)
  line L33 (7.1376, 13.2315, -0.5425) -> (7.1376, 106.6129, -0.5425)
  line L34 (77.6309, 49.5898, -0.5425) -> (106.5409, 39.6147, -0.5425)
  line L35 (85.3097, 78.7939, -0.5425) -> (105.004, 76.458, -0.5425)
  line L36 (103.6411, 42.6291, -0.5425) -> (75.7593, 52.1381, -0.5425)
  arc A28 through (13.5344, 101.8013, -0.5425) (11.1356, 100.8077, -0.5425) (10.1419, 98.4088, -0.5425)
  line L37 (37.6621, 101.8013, -0.5425) -> (13.5344, 101.8013, -0.5425)
  arc A29 through (68.665, 71.0412, -0.5425) (66.7178, 68.5186, -0.5425) (66.9703, 65.342, -0.5425)
  arc A30 through (71.4916, 55.926, -0.5425) (73.2442, 53.6025, -0.5425) (75.7593, 52.1381, -0.5425)
  line L38 (68.665, 71.0412, -0.5425) -> (79.3035, 77.4917, -0.5425)
  line L39 (71.4916, 55.926, -0.5425) -> (66.9703, 65.342, -0.5425)
  arc A31 through (10.1419, 89.8693, -0.5425) (10.8294, 87.7729, -0.5425) (12.6248, 86.4908, -0.5425)
  line L40 (88.0477, 102.9769, -0.5425) -> (83.9707, 85.1234, -0.5425)
  line L41 (61.4337, 69.0534, -0.5425) -> (13.9723, 83.8929, -0.5425)
  arc A32 through (85.4902, 101.6133, -0.5425) (84.7499, 104.858, -0.5425) (81.7514, 106.3021, -0.5425)
  line L42 (3.4675, 5.4848, -0.5425) -> (3.4675, 115.3458, -0.5425)
  arc A33 through (198.0965, 82.5311, -0.5425) (195.738, 80.6968, -0.5425) (196.1913, 77.7435, -0.5425)
  arc A34 through (85.3097, 78.7939, -0.5425) (82.1977, 78.6452, -0.5425) (79.3035, 77.4917, -0.5425)
  arc A35 through (77.6309, 49.5898, -0.5425) (73.9232, 49.2086, -0.5425) (71.8221, 46.13, -0.5425)
  line L43 (81.1941, 82.8007, -0.5425) -> (85.4902, 101.6133, -0.5425)
  line L44 (53.0443, 13.4172, -0.5425) -> (61.1239, 13.4172, -0.5425)
  arc A36 through (13.9723, 83.8929, -0.5425) (11.3447, 83.4543, -0.5425) (10.1419, 81.0774, -0.5425)
  arc A37 through (10.1419, 17.1047, -0.5425) (11.222, 14.4972, -0.5425) (13.8294, 13.4172, -0.5425)
  arc A38 through (107.9965, 73.0335, -0.5425) (107.159, 75.3214, -0.5425) (105.004, 76.458, -0.5425)
  line L45 (45.4146, 19.1097, -0.5425) -> (15.5677, 65.1774, -0.5425)
  line L46 (12.6248, 86.4908, -0.5425) -> (62.0516, 71.0259, -0.5425)
  arc A39 through (197.4845, 37.6248, -0.5425) (196.6144, 39.4665, -0.5425) (194.7583, 40.3053, -0.5425)
  line L47 (188.6375, 13.4172, -0.5425) -> (196.4178, 13.4172, -0.5425)
  arc A40 through (287.9958, 78.9742, -0.5425) (291.7741, 79.7965, -0.5425) (293.4635, 83.2746, -0.5425)
  line L48 (13.8294, 13.4172, -0.5425) -> (42.3199, 13.4172, -0.5425)
  arc A41 through (50.5643, 14.7697, -0.5425) (51.6319, 13.7773, -0.5425) (53.0443, 13.4172, -0.5425)
  line L49 (152.619, 55.5584, -0.5425) -> (176.2747, 86.6068, -0.5425)
  line L50 (156.4587, 57.3551, -0.5425) -> (176.5219, 83.9467, -0.5425)
  arc A42 through (272.2404, 84.6401, -0.5425) (272.9897, 83.1158, -0.5425) (274.4552, 82.2574, -0.5425)
  arc A43 through (7.1376, 13.2315, -0.5425) (7.7856, 11.667, -0.5425) (9.3501, 11.019, -0.5425)
  line L51 (187.1226, 79.6326, -0.5425) -> (194.4335, 46.3539, -0.5425)
  line L52 (236.1917, 94.9829, -0.5425) -> (264.0999, 86.0696, -0.5425)
  line L53 (147.6751, 50.636, -0.5425) -> (116.5331, 74.4839, -0.5425)
  arc A44 through (235.2375, 65.7635, -0.5425) (236.4809, 64.4222, -0.5425) (238.1606, 63.6983, -0.5425)
  arc A45 through (256.0736, 62.249, -0.5425) (254.4848, 59.4332, -0.5425) (254.2531, 56.2083, -0.5425)
  arc A46 through (15.5677, 65.1774, -0.5425) (12.2556, 66.4023, -0.5425) (10.1419, 63.5734, -0.5425)
  arc A47 through (265.809, 81.0232, -0.5425) (265.0201, 83.0079, -0.5425) (263.2633, 84.2224, -0.5425)
  arc A48 through (236.9767, 92.6733, -0.5425) (234.4712, 92.5836, -0.5425) (232.6022, 90.9126, -0.5425)
  arc A49 through (62.0516, 71.0259, -0.5425) (63.5927, 70.8841, -0.5425) (65.0563, 71.387, -0.5425)
  arc A50 through (232.5299, 15.7176, -0.5425) (234.1555, 14.0355, -0.5425) (236.4115, 13.4172, -0.5425)
  arc A51 through (264.0999, 86.0696, -0.5425) (267.6144, 86.7764, -0.5425) (268.8676, 90.1351, -0.5425)
  line L54 (123.5394, 72.2398, -0.5425) -> (146.4088, 54.7269, -0.5425)
  line L55 (64.7618, 16.502, -0.5425) -> (70.492, 51.0906, -0.5425)
  line L56 (236.9767, 92.6733, -0.5425) -> (263.2633, 84.2224, -0.5425)
  line L57 (182.035, 85.2385, -0.5425) -> (183.2206, 84.6451, -0.5425)
  arc A52 through (277.0376, 79.3533, -0.5425) (272.8243, 79.1546, -0.5425) (269.2803, 76.8674, -0.5425)
  arc A53 through (9.3501, 108.8254, -0.5425) (7.7856, 108.1774, -0.5425) (7.1376, 106.6129, -0.5425)
  line L58 (10.1419, 63.5734, -0.5425) -> (10.1419, 17.1047, -0.5425)
  line L59 (131.7372, 20.1938, -0.5425) -> (148.5132, 45.6809, -0.5425)
  arc A54 through (293.4635, 101.8771, -0.5425) (292.1675, 105.006, -0.5425) (289.0385, 106.3021, -0.5425)
  line L60 (153.5813, 49.6685, -0.5425) -> (133.0891, 17.9687, -0.5425)
  line L61 (275.8299, 33.4326, -0.5425) -> (292.1232, 53.2736, -0.5425)
  line L62 (269.4929, 101.1507, -0.5425) -> (272.2404, 84.6401, -0.5425)
  arc A55 through (61.1239, 13.4172, -0.5425) (63.5088, 14.2922, -0.5425) (64.7618, 16.502, -0.5425)
  line L63 (173.0748, 45.173, -0.5425) -> (157.4975, 52.9381, -0.5425)
  line L64 (296.5336, 106.6129, -0.5425) -> (296.5336, 13.2315, -0.5425)
  arc A56 through (293.4635, 72.1916, -0.5425) (292.4863, 74.9652, -0.5425) (289.9863, 76.5139, -0.5425)
  arc A57 through (10.1419, 79.0457, -0.5425) (10.3518, 77.5888, -0.5425) (10.9643, 76.2502, -0.5425)
  line L65 (10.1419, 81.0774, -0.5425) -> (10.1419, 79.0457, -0.5425)
  line L66 (262.6115, 106.3021, -0.5425) -> (235.8049, 106.3021, -0.5425)
  line L67 (254.2531, 56.2083, -0.5425) -> (258.1218, 30.4824, -0.5425)
  arc A58 through (123.6315, 13.4172, -0.5425) (126.3137, 15.139, -0.5425) (125.8648, 18.2946, -0.5425)
  arc A59 through (182.035, 85.2385, -0.5425) (179.0447, 85.5899, -0.5425) (176.5219, 83.9467, -0.5425)
  arc A60 through (148.5132, 45.6809, -0.5425) (149.0689, 48.3233, -0.5425) (147.6751, 50.636, -0.5425)
  line L68 (120.1949, 80.8795, -0.5425) -> (123.35, 102.0715, -0.5425)
  line L69 (196.1913, 77.7435, -0.5425) -> (213.8317, 56.0762, -0.5425)
  line L70 (217.428, 55.2949, -0.5425) -> (231.2263, 62.1248, -0.5425)
  arc A61 through (187.1226, 79.6326, -0.5425) (185.7389, 82.5805, -0.5425) (183.2206, 84.6451, -0.5425)
  arc A62 through (239.2829, 61.3876, -0.5425) (235.7303, 61.4569, -0.5425) (232.339, 60.3964, -0.5425)
  arc A63 through (173.0748, 45.173, -0.5425) (175.7805, 44.1418, -0.5425) (178.6355, 43.6591, -0.5425)
  line L71 (194.7583, 40.3053, -0.5425) -> (181.0984, 41.2901, -0.5425)
  line L72 (191.3482, 42.778, -0.5425) -> (178.6355, 43.6591, -0.5425)
  line L73 (172.3385, 106.3021, -0.5425) -> (128.5492, 106.3021, -0.5425)
  arc A64 through (175.2618, 103.748, -0.5425) (174.2794, 105.5736, -0.5425) (172.3385, 106.3021, -0.5425)
  arc A65 through (191.3482, 42.778, -0.5425) (193.7858, 43.7939, -0.5425) (194.4335, 46.3539, -0.5425)
  arc A66 through (156.4587, 57.3551, -0.5425) (155.942, 54.9029, -0.5425) (157.4975, 52.9381, -0.5425)
  line L74 (135.5665, 13.4172, -0.5425) -> (180.1276, 13.4172, -0.5425)
  line L75 (180.9121, 87.7982, -0.5425) -> (188.1391, 84.5978, -0.5425)
  arc A67 through (176.2747, 86.6068, -0.5425) (177.0332, 88.1586, -0.5425) (177.1399, 89.8825, -0.5425)
  arc A68 through (146.4088, 54.7269, -0.5425) (149.6864, 53.8542, -0.5425) (152.619, 55.5584, -0.5425)
  line L76 (171.2495, 43.7449, -0.5425) -> (157.3818, 50.7036, -0.5425)
  arc A69 through (115.2719, 77.1399, -0.5425) (118.4948, 78.0074, -0.5425) (120.1949, 80.8795, -0.5425)
  line L77 (256.3019, 29.2016, -0.5425) -> (252.4432, 55.9167, -0.5425)
  line L78 (215.0822, 98.9802, -0.5425) -> (209.3714, 105.3255, -0.5425)
  arc A70 through (213.8317, 56.0762, -0.5425) (215.4931, 55.056, -0.5425) (217.428, 55.2949, -0.5425)
  arc A71 through (180.1276, 13.4172, -0.5425) (182.5336, 14.6603, -0.5425) (182.9119, 17.342, -0.5425)
  line L79 (226.4521, 101.7184, -0.5425) -> (220.6389, 98.3761, -0.5425)
  arc A72 through (123.35, 102.0715, -0.5425) (122.4956, 105.0224, -0.5425) (119.7027, 106.3021, -0.5425)
  arc A73 through (252.4432, 55.9167, -0.5425) (251.2505, 58.3541, -0.5425) (248.8594, 59.637, -0.5425)
  line L80 (182.9119, 17.342, -0.5425) -> (175.2679, 39.1748, -0.5425)
  line L81 (300.5325, 115.3458, -0.5425) -> (300.5325, 5.4848, -0.5425)
  arc A74 through (180.3167, 106.3021, -0.5425) (178.0915, 105.2889, -0.5425) (177.3948, 102.9453, -0.5425)
  line L82 (232.3424, 101.3464, -0.5425) -> (233.851, 97.2274, -0.5425)
  line L83 (212.3403, 54.5979, -0.5425) -> (195.9237, 74.8489, -0.5425)
  arc A75 through (188.1391, 84.5978, -0.5425) (191.1487, 83.7484, -0.5425) (194.2757, 83.7751, -0.5425)
  arc A76 through (181.0984, 41.2901, -0.5425) (178.5412, 40.1374, -0.5425) (178.1042, 37.3666, -0.5425)
  line L84 (228.1101, 82.5801, -0.5425) -> (232.6022, 90.9126, -0.5425)
  line L85 (125.6327, 103.7957, -0.5425) -> (121.5744, 77.1149, -0.5425)
  arc A77 through (175.2679, 39.1748, -0.5425) (173.7034, 41.8509, -0.5425) (171.2495, 43.7449, -0.5425)
  line L86 (177.1399, 89.8825, -0.5425) -> (175.2618, 103.748, -0.5425)
  arc A78 through (157.3818, 50.7036, -0.5425) (155.2835, 50.9132, -0.5425) (153.5813, 49.6685, -0.5425)
  line L87 (293.4635, 83.2746, -0.5425) -> (293.4635, 101.8771, -0.5425)
  line L88 (289.9863, 76.5139, -0.5425) -> (277.0376, 79.3533, -0.5425)
  line L89 (265.809, 81.0232, -0.5425) -> (265.9528, 79.3271, -0.5425)
  line L90 (177.3948, 102.9453, -0.5425) -> (179.1848, 90.0888, -0.5425)
  arc A79 through (185.8555, 15.3861, -0.5425) (186.9334, 13.9592, -0.5425) (188.6375, 13.4172, -0.5425)
  arc A80 through (249.4163, 61.4315, -0.5425) (252.1126, 61.6099, -0.5425) (254.3494, 63.126, -0.5425)
  arc A81 through (128.5492, 106.3021, -0.5425) (126.6265, 105.5894, -0.5425) (125.6327, 103.7957, -0.5425)
  arc A82 through (133.0891, 17.9687, -0.5425) (132.9755, 14.9568, -0.5425) (135.5665, 13.4172, -0.5425)
  arc A83 through (121.5744, 77.1149, -0.5425) (121.89, 74.4085, -0.5425) (123.5394, 72.2398, -0.5425)
  arc A84 through (179.1848, 90.0888, -0.5425) (179.7513, 88.7194, -0.5425) (180.9121, 87.7982, -0.5425)
  line L91 (204.6745, 13.4172, -0.5425) -> (226.6063, 13.4172, -0.5425)
  line L92 (249.4163, 61.4315, -0.5425) -> (238.1606, 63.6983, -0.5425)
  arc A85 through (127.0398, 19.8883, -0.5425) (129.4645, 18.872, -0.5425) (131.7372, 20.1938, -0.5425)
  line L93 (264.5468, 74.9815, -0.5425) -> (254.3494, 63.126, -0.5425)
  line L94 (178.1042, 37.3666, -0.5425) -> (185.8555, 15.3861, -0.5425)
  arc A86 through (230.7073, 100.1344, -0.5425) (228.9517, 101.9257, -0.5425) (226.4521, 101.7184, -0.5425)
  line L95 (289.0385, 106.3021, -0.5425) -> (273.8579, 106.3021, -0.5425)
  arc A87 through (196.7325, 45.5183, -0.5425) (198.3819, 43.4786, -0.5425) (201.0039, 43.5591, -0.5425)
  arc A88 through (266.9865, 102.5405, -0.5425) (265.4964, 105.2324, -0.5425) (262.6115, 106.3021, -0.5425)
  arc A89 through (213.4569, 83.3852, -0.5425) (211.0714, 83.9348, -0.5425) (208.6237, 83.9074, -0.5425)
  arc A90 through (201.6545, 41.8242, -0.5425) (199.8127, 39.9794, -0.5425) (199.3291, 37.4177, -0.5425)
  arc A91 through (264.5468, 74.9815, -0.5425) (265.6874, 77.0128, -0.5425) (265.9528, 79.3271, -0.5425)
  line L96 (248.8594, 59.637, -0.5425) -> (239.2829, 61.3876, -0.5425)
  line L97 (269.2803, 76.8674, -0.5425) -> (256.0736, 62.249, -0.5425)
  arc A92 through (220.6389, 98.3761, -0.5425) (218.6659, 96.8329, -0.5425) (217.2044, 94.7987, -0.5425)
  arc A93 through (228.1101, 82.5801, -0.5425) (227.4932, 80.0143, -0.5425) (228.2248, 77.4788, -0.5425)
  arc A94 through (214.0829, 45.1294, -0.5425) (212.3427, 46.53, -0.5425) (210.1198, 46.3093, -0.5425)
  arc A95 through (226.6063, 13.4172, -0.5425) (229.1471, 14.8682, -0.5425) (229.1883, 17.794, -0.5425)
  arc A96 through (230.7717, 91.8438, -0.5425) (231.7374, 95.0695, -0.5425) (231.3102, 98.4094, -0.5425)
  arc A97 through (226.309, 76.7604, -0.5425) (224.4925, 78.8998, -0.5425) (222.0557, 80.2922, -0.5425)
  line L98 (199.3562, 16.6291, -0.5425) -> (197.4845, 37.6248, -0.5425)